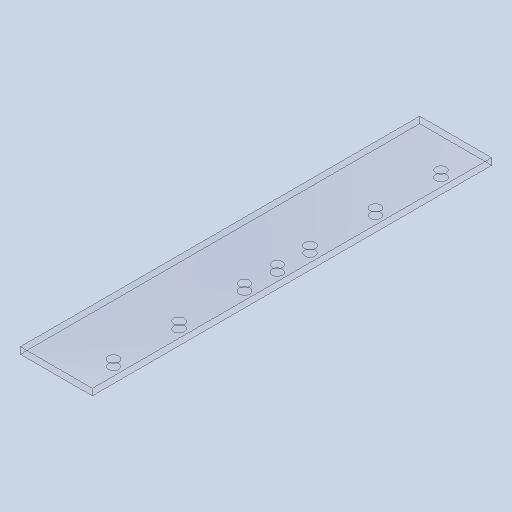
# Autodesk Inventor part: sensorPCB
Saved by Autodesk Inventor 2022 (Build 260153000, 153)
## iProperties
Created: 2021-07-08
Part Number: sensorPCB
Material: エポキシ樹脂
Document SubType Name: Modeling
Designer: ken
Density: 1.14 g/cm^3
Appearance: 透明 - スレート 青
Mass: 5.99116 g
Surface Area: 59.7215 cm^2
Volume: 5.25541 cm^3
Author: ken
Autodesk Inventor part; units mm, degrees
ref_plane "YZ Plane" through (0, 0, 0) normal (1, 0, 0) x (0, 1, 0)
ref_plane "XZ Plane" through (0, 0, 0) normal (0, 1, 0) x (-1, 0, 0)
ref_plane "XY Plane" through (0, 0, 0) normal (0, 0, 1) x (1, 0, 0)
sketch "スケッチ1" plane through (0, 0, 0) normal (0, 1, 0) x (-1, 0, 0)
  line L0 (0, 0) -> (22, 0)
  line L1 (22, 0) -> (22, -122)
  line L2 (22, -122) -> (0, -122)
  line L3 (0, -122) -> (0, 0)
  dimension "d0" = 22
  dimension "d1" = 122
  constraints: 8 end point, 2 parallel, 1 horizontal, 1 perpendicular
  measures "d0" distance of L1.end L2.end
  measures "d1" distance of L0.end L1.end
extrude "押し出し1" add sketch "スケッチ1" along normal blind 2
sketch "スケッチ2" plane through (0, 2, 0) normal (0, 1, 0) x (1, 0, 0)
  line L0 (0, 0) -> (0, 122) projected
  line L1 (-22, 0) -> (0, 0) projected
  line L2 (0, 122) -> (-22, 122) projected
  point P0 (-4.5, 11)
  point P1 (-4.5, 31)
  point P2 (-4.5, 51)
  point P3 (-4.5, 61)
  point P4 (-4.5, 71)
  point P5 (-4.5, 91)
  point P6 (-4.5, 111)
  dimension "d13" = 4.5
  dimension "d14" = 20
  dimension "d16" = 11
  dimension "d17" = 20
  dimension "d18" = 10
  dimension "d19" = 10
  dimension "d20" = 20
  dimension "d21" = 20
  dimension "d22" = 11
  constraints: 6 vertical alignment
  measures "d13" distance from line of L0 point (-4.5, 11)
  measures "d14" distance of point (-4.5, 31) point (-4.5, 11)
  measures "d16" distance from line of L1 point (-4.5, 11)
  measures "d17" distance of point (-4.5, 51) point (-4.5, 31)
  measures "d18" distance of point (-4.5, 51) point (-4.5, 61)
  measures "d19" distance of point (-4.5, 61) point (-4.5, 71)
  measures "d20" distance of point (-4.5, 71) point (-4.5, 91)
  measures "d21" distance of point (-4.5, 91) point (-4.5, 111)
  measures "d22" distance from line of L2 point (-4.5, 111)
hole "穴1" at (-4.5, 2, -11) at (-4.5, 2, -31) at (-4.5, 2, -51) at (-4.5, 2, -61) at (-4.5, 2, -71) at (-4.5, 2, -91) at (-4.5, 2, -111) direction (0, -1, 0) diameter 3.2 depth 3
